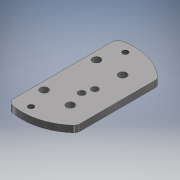
# Autodesk Inventor part: Shield_3_Ground_v4
Saved by Autodesk Inventor 2018 (Build 220112000, 112)
## iProperties
Created: 2015-02-10
Part Number: Shield_3_Ground_v4
Material: Stainless Steel
Document SubType Name: Modeling
Designer: Pascal
Density: 8 g/cm^3
Appearance: Stainless - Brushed
Author: Pascal
Autodesk Inventor part; units mm, degrees
ref_plane "YZ Plane" through (0, 0, 0) normal (1, 0, 0) x (0, 1, 0)
ref_plane "XZ Plane" through (0, 0, 0) normal (0, 1, 0) x (-1, 0, 0)
ref_plane "XY Plane" through (0, 0, 0) normal (0, 0, 1) x (1, 0, 0)
sketch "Sketch1" plane through (0, 0, 0) normal (0, 1, 0) x (-1, 0, 0)
  circle A0 centre (0, 0) radius 27.305
  dimension "d85" = 54.61
  constraints: 1 centre point, 1 coincident
  measures "d85" diameter of A0
extrude "Extrusion1" add sketch "Sketch1" along normal blind 3.175
sketch "Sketch2" plane through (0, 3.175, 0) normal (0, 1, 0) x (1, 0, 0)
  circle A0 centre (0, -22.86) radius 1.905
  circle A1 centre (0, 22.86) radius 1.905
  circle A2 centre (0, 0) radius 3.4925
  circle A3 centre (0, 0) radius 27.305 projected
  line L0 (0, 0) -> (0, -35.2816) construction
  line L1 (0, 0) -> (-33.3398, 0) construction
  circle A4 centre (0, -22.86) radius 4.7625
  dimension "d105" = 6.985
  dimension "d107" = 3.81
  dimension "d109" = 3.81
  dimension "d147" = 0
  dimension "d148" = 0
  dimension "d149" = 22.86
  dimension "d150" = 22.86
  dimension "d151" = 9.525
  constraints: 4 centre point, 4 end point, 2 coincident, 1 horizontal, 1 vertical
  measures "d105" diameter of A2
  measures "d107" diameter of A1
  measures "d109" diameter of A0
  measures "d147" distance from line of A0.centre L0
  measures "d148" distance from line of L0 A1.centre
  measures "d149" distance from line of L1 A0.centre
  measures "d150" distance from line of L1 A1.centre
  measures "d151" diameter of A4
sketch "Sketch3" plane through (0, 0, 0) normal (0, -1, 0) x (1, 0, 0)
  line L0 (-12.7, -4.445) -> (-2.54, -4.445)
  line L1 (-2.54, -4.445) -> (-2.54, 4.445)
  line L2 (-2.54, 4.445) -> (-12.7, 4.445)
  line L3 (-12.7, 4.445) -> (-12.7, -4.445)
  line L4 (-38.227, 0) -> (38.227, 0) projected
  line L5 (0, -38.227) -> (0, 38.227) projected
  point P0 (0, 0)
  dimension "d116" = 10.16
  dimension "d125" = 8.89
  dimension "d126" = 12.7
  constraints: 8 end point, 2 parallel, 1 horizontal, 1 perpendicular, 1 other
  measures "d116" distance between parallel lines of L1 L3
  measures "d125" distance of L0.end L1.end
  measures "d126" distance between parallel lines of L5 L3
extrude "Extrusion3" [suppressed]
fillet "Fillet1" [suppressed]
sketch "Sketch4" plane through (0, 3.175, 0) normal (0, 1, 0) x (1, 0, 0)
  circle A0 centre (0, 0) radius 27.305 projected
  line L0 (-7.62, -26.2202) -> (-7.62, 26.2202)
  line L1 (19.05, -19.5617) -> (19.05, 19.5617)
  dimension "d121" = 7.62
  dimension "d122" = 19.05
  constraints: 4 end point, 4 point on circle, 2 vertical
  measures "d121" distance from line of point (0, 0) L0
  measures "d122" distance from line of point (0, 0) L1
extrude "Extrusion4" cut sketch "Sketch4" against normal through all contours A0 L1 | L0 A0
hole "Hole10" at (0, 3.175, -22.86) at (0, 3.175, 22.86) direction (0, -1, 0) diameter 2.6416 end through all thread size "6-32 UNC" class "2B" standard "ANSI Unified Screw Threads"
sketch "Sketch5" plane through (0, 3.175, 0) normal (0, 1, 0) x (1, 0, 0)
  line L0 (0, 0) -> (23.5566, 0) construction
  line L1 (19.05, -19.5617) -> (19.05, 19.5617) projected
  point P0 (8.89, 12.6873)
  point P1 (8.89, -12.6873)
  point P2 (-3.81, -12.6873)
  point P3 (-3.81, 12.6873)
  dimension "d136" = 25.3746
  dimension "d137" = 12.7
  dimension "d146" = 22.86
  dimension "d160" = 22.86
  dimension "d161" = 10.16
  constraints: 2 end point, 2 symmetric about line, 1 horizontal
  measures "d136" distance of point (-3.81, -12.687) point (-3.81, 12.687)
  measures "d137" distance of point (8.89, 12.687) point (-3.81, 12.687)
  measures "d146" distance from line of point (-3.81, 12.687) L1
  measures "d160" distance from line of L1 point (-3.81, -12.687)
  measures "d161" distance from line of L1 point (8.89, -12.687)
hole "Hole11" at (8.89, 3.175, -12.6873) at (8.89, 3.175, 12.6873) at (-3.81, 3.175, 12.6873) at (-3.81, 3.175, -12.6873) direction (0, -1, 0) diameter 3.81 depth 25.4 tip angle 118 clearance for "Flat Head Machine Screw (82)" size "#6" standard "Ansi Unified Screw Threads"
sketch "Sketch6" plane through (0, 0, 0) normal (0, -1, 0) x (1, 0, 0)
  circle A0 centre (8.1279, 0.0315) radius 1.5875 projected
  circle A1 centre (6.5218, 4.8509) radius 1.5875 projected
  circle A2 centre (8.1279, 0.0315) radius 1.5875 projected
  line L0 (-0.8446, 5.1702) -> (-2.5619, 10.3231) projected
  arc A3 (4.1433, -9.7961) -> (-2.5619, 10.3231) centre (0, 0) ccw projected
  line L1 (4.1433, -9.7961) -> (2.426, -4.6432) projected
  arc A4 (2.426, -4.6432) -> (-0.8446, 5.1702) centre (0, 0) ccw projected
  point P0 (0, 0)
  constraints: 2 coincident
hole "Hole12" at (8.1279, 0, 0.0315) at (6.5218, 0, 4.8509) direction (0, 1, 0) diameter 3.175 end through all
fillet "Fillet2" radius 3.175 4 edges at (-7.62, 1.5875, 26.2202) (-7.62, 1.5875, -26.2202) (19.05, 1.5875, 19.5617) (19.05, 1.5875, -19.5617)
equation "\"d107\" = d106"
equation "\"d109\" = d106"
equation "\"d150\" = d149"
equation "\"d106\" = 3.81"
body "Solid1"
